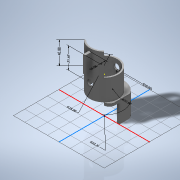
# Autodesk Inventor part: Part1
Saved by Autodesk Inventor 2022 (Build 260153000, 153)
## iProperties
Created: 2021-09-21
Part Number: Part1
Material: Generic
Document SubType Name: Modeling
Designer: WASHINGTON
Density: 1 g/cm^3
Appearance: Default
Author: WASHINGTON
Autodesk Inventor part; units mm, degrees
ref_plane "YZ Plane" through (0, 0, 0) normal (1, 0, 0) x (0, 1, 0)
ref_plane "XZ Plane" through (0, 0, 0) normal (0, 1, 0) x (-1, 0, 0)
sketch "Sketch1" plane through (0, 0, 0) normal (0, 1, 0) x (-1, 0, 0)
  circle A0 centre (0, 0) radius 20.5
  circle A1 centre (0, 0) radius 25
  dimension "d0" = 41
  dimension "d1" = 50
  constraints: 2 centre point, 2 coincident
  measures "d0" diameter of A0
  measures "d1" diameter of A1
extrude "Extrusion1" add sketch "Sketch1" along normal blind 12.5 and the other way blind 25
sketch "Sketch2" plane through (0, 0, 0) normal (0, 0, 1) x (1, 0, 0)
  circle A0 centre (0, 0) radius 5
  dimension "d4" = 10
  constraints: 1 centre point, 1 coincident
  measures "d4" diameter of A0
extrude "Extrusion2" cut sketch "Sketch2" along normal through all both and the other way through all
sketch "Sketch3" plane through (0, -25, 0) normal (0, -1, 0) x (1, 0, 0)
  arc A0 (23.5516, -23.5516) -> (23.5516, 23.5516) centre (0, 0) ccw
  line L0 (0, 0) -> (23.5516, 23.5516) construction
  line L1 (0, 0) -> (33.307, 0) construction
  line L2 (0, 0) -> (23.5516, -23.5516) construction
  circle A1 centre (0, 0) radius 25 construction
  circle A2 centre (0, 0) radius 20.5 construction
  arc A3 (14.4957, -14.4957) -> (14.4957, 14.4957) centre (0, 0) ccw
  line L3 (14.4957, 14.4957) -> (23.5516, 23.5516)
  line L4 (0.0405, -20.5) -> (0.0405, -33.307)
  arc A4 (0.0405, -33.307) -> (23.5516, -23.5516) centre (0, 0) ccw
  arc A5 (0.0405, -20.5) -> (14.4957, -14.4957) centre (0, 0) ccw
  dimension "d7" = 33.307
  dimension "d8" = 45
  dimension "d9" = 90
  dimension "d26" = 12.807
  constraints: 11 point on circle, 10 end point, 4 centre point, 4 coincident, 1 collinear, 1 equal length, 1 horizontal, 1 vertical, 1 other
  measures "d7" radius of A0
  measures "d8" angle of L1 L0
  measures "d9" angle of L2 L0
  measures "d26" distance of L4.start L4.end
extrude "Extrusion3" add sketch "Sketch3" along normal blind 5
sketch "Sketch6" plane through (0, -30, 0) normal (0, -1, 0) x (1, 0, 0)
  arc A0 (0.0405, -20.5) -> (14.4957, 14.4957) centre (0, 0) ccw projected
  line L0 (8.0405, -18.8574) -> (8.0405, -28)
  line L1 (8.0405, -28) -> (0.0405, -28)
  line L2 (0.0405, -28) -> (0.0405, -20.5)
  line L3 (0.0405, -25) -> (0.0405, -20.5) projected
  arc A1 (0.0405, -20.5) -> (8.0405, -18.8574) centre (0, 0) ccw
  dimension "d14" = 8
  dimension "d15" = 42.4957
  constraints: 6 end point, 3 point on circle, 2 parallel, 1 centre point, 1 coincident, 1 horizontal
  measures "d14" distance of L0.end L1.end
  measures "d15" distance from line of A0.end L1
extrude "Extrusion4" add sketch "Sketch6" along normal blind 5
sketch "Sketch7" plane through (0, -30, 0) normal (0, -1, 0) x (1, 0, 0)
  line L0 (0.0405, -28) -> (8.0381, -28) projected
  line L1 (8.0381, -28) -> (18.0381, -28)
  line L2 (18.0381, -28) -> (18.0381, -9.7405)
  line L3 (8.0381, -18.8584) -> (8.0381, -28)
  circle A0 centre (0, 0) radius 20.5
  arc A1 (18.0381, -28) -> (33.3072, 0) centre (0, 0) ccw
  line L4 (33.3072, 0) -> (20.5, 0)
  circle A2 centre (0, 0) radius 20.5 projected
  point P0 (0.0405, -33.307)
  point P1 (8.0405, -18.8574)
  point P2 (8.0381, -18.8584)
  dimension "d19" = 10
  dimension "d22" = 41
  dimension "d23" = 28
  dimension "d24" = 28
  dimension "d25" = 2.4619
  constraints: 6 end point, 5 point on circle, 2 centre point, 2 coincident, 2 horizontal, 1 perpendicular, 1 vertical, 4 other
  measures "d22" diameter of A0
  measures "d23" distance between parallel lines of L4 L0
  measures "d24" distance from line of point (20.5, 0) L0
  measures "d25" distance from line of point (20.5, 0) L2
extrude "Extrusion5" add sketch "Sketch7" along normal blind 23 contours L2 A0 L4 A1
sketch "Sketch8" plane through (8.0405, -30, -28) normal (0, 0, -1) x (-1, 0, 0)
  line L0 (8, -5) -> (0, -5) projected
  line L1 (0, 0) -> (8, 0) projected
  line L2 (8, -5) -> (0, -5)
  line L3 (0, -5) -> (0, 0)
  line L4 (0, 0) -> (8, 0)
  line L5 (8, 0) -> (8, -5)
  point P0 (8.0405, 30)
  constraints: 8 end point, 2 parallel, 1 horizontal, 1 perpendicular
extrude "Extrusion6" add sketch "Sketch8" along normal up to surface round surface about axis through (0, -25, 0) along (0, -1, 0) radius 33.307 far side no
sketch "Sketch9" plane through (0, -53, 0) normal (0, -1, 0) x (1, 0, 0)
  line L0 (0.0405, -25) -> (0.0405, -33.307) projected
  line L1 (0.0405, -33.307) -> (8.0405, -33.307)
  line L2 (8.0405, -33.307) -> (8.0405, -18.8574)
  line L3 (8.0405, -18.8574) -> (0.0405, -18.8574)
  line L4 (0.0405, -18.8574) -> (0.0405, -33.307)
  point P0 (0, 0)
  constraints: 8 end point, 2 parallel, 1 horizontal, 1 perpendicular
extrude "Extrusion7" add sketch "Sketch9" along normal blind 5
sketch "Sketch10" plane through (0, -53, 0) normal (0, -1, 0) x (1, 0, 0)
  line L0 (0.0405, -33.307) -> (8.0405, -33.307) projected
  arc A0 (0.0405, -33.307) -> (23.5516, 23.5516) centre (0, 0) ccw projected
  arc A1 (0.0405, -33.307) -> (33.3068, 0.1051) centre (0, 0) ccw
  line L1 (33.3068, 0.1051) -> (56.6736, 0.1051)
  line L2 (56.6736, 0.1051) -> (0.0405, -55.1449)
  line L3 (0.0405, -55.1449) -> (0.0405, -33.307)
  dimension "d31" = 135.708
  dimension "d32" = 33.4121
  dimension "d33" = 39.9123
  constraints: 6 end point, 3 point on circle, 1 centre point, 1 coincident, 1 horizontal, 1 perpendicular
  measures "d31" angle of L0 L2
  measures "d32" distance between parallel lines of L0 L1
  measures "d33" distance from line of A0.end L2
extrude "Extrusion8" cut sketch "Sketch10" along normal blind 5
sketch "Sketch11" plane through (0, -53, 0) normal (0, -1, 0) x (1, 0, 0)
  arc A0 (0.0405, -33.307) -> (8.0405, -32.3219) centre (0, 0) ccw projected
  line L0 (20.5, 0) -> (33.307, 0) projected
  arc A1 (0.0405, -33.307) -> (33.307, 0) centre (0, 0) ccw
  circle A2 centre (0, 0) radius 20.5 projected
  arc A3 (0.0405, -20.5) -> (20.5, 0) centre (0, 0) ccw
  line L1 (33.307, 0) -> (20.5, 0)
  line L2 (0.0405, -25) -> (0.0405, -33.307) projected
  line L3 (0.0405, -33.307) -> (0.0405, -20.5)
  point P0 (8.0405, -32.3219)
  constraints: 5 point on circle, 4 end point, 2 centre point, 2 coincident, 2 collinear
extrude "Extrusion9" add sketch "Sketch11" along normal blind 5 contours L2 L3 A2 L0 A1 A0
sketch "Sketch12" plane through (0, 0, 0) normal (0, 1, 0) x (-1, 0, 0)
  point P0 (0, 0)
extrude "Extrusion10" cut sketch "Sketch11" along normal blind 5 contours A2
sketch "Sketch13" plane through (0, -58, 0) normal (0, -1, 0) x (1, 0, 0)
  arc A0 (0.0405, -33.307) -> (33.307, 0) centre (0, 0) ccw projected
  line L0 (0.0405, -33.307) -> (0.0405, -20.5)
  line L1 (18.0381, -9.7405) -> (18.0381, -27.9997) projected
  line L2 (18.0381, -27.9997) -> (18.0381, -9.7405)
  arc A1 (0.0405, -20.5) -> (18.0381, -9.7405) centre (0, 0) ccw projected
  arc A2 (0.0405, -20.5) -> (18.0381, -9.7405) centre (0, 0) ccw
  arc A3 (0.0405, -33.307) -> (18.0381, -27.9997) centre (0, 0) ccw projected
  arc A4 (0.0405, -33.307) -> (18.0381, -27.9997) centre (0, 0) ccw
  constraints: 5 point on circle, 4 end point, 2 centre point, 2 coincident, 1 vertical
extrude "Extrusion11" cut sketch "Sketch13" against normal blind 5
sketch "Sketch14" plane through (0, -58, 0) normal (0, -1, 0) x (1, 0, 0)
  line L0 (0.0405, -25) -> (0.0405, -33.307) projected
  line L1 (0.0405, -33.307) -> (0.0405, -20.5)
  circle A0 centre (0, 0) radius 20.5 projected
  line L2 (8.0405, -18.8574) -> (8.0405, -32.3219) projected
  line L3 (8.0405, -32.3219) -> (8.0405, -18.8574)
  arc A1 (0.0405, -20.5) -> (8.0405, -18.8574) centre (0, 0) ccw projected
  arc A2 (8.0405, -18.8574) -> (18.0381, -9.7405) centre (0, 0) ccw projected
  arc A3 (0.0405, -20.5) -> (8.0405, -18.8574) centre (0, 0) ccw
  arc A4 (0.0405, -33.307) -> (8.0405, -32.3219) centre (0, 0) ccw
  constraints: 5 point on circle, 4 end point, 2 centre point, 2 coincident, 1 collinear, 1 vertical
extrude "Extrusion12" add sketch "Sketch14" along normal blind 5 contours L1 A0 L2 A4 L0
sketch "Sketch15" plane through (0, -58, 0) normal (0, -1, 0) x (1, 0, 0)
  line L0 (33.307, 0) -> (20.5, 0) projected
  line L1 (33.307, 0) -> (20.5, 0)
  circle A0 centre (0, 0) radius 20.5 projected
  line L2 (8.0405, -32.3219) -> (8.0405, -18.8574) projected
  line L3 (8.0405, -32.3219) -> (8.0405, -18.8574)
  arc A1 (0.0405, -20.5) -> (8.0405, -18.8574) centre (0, 0) ccw projected
  arc A2 (8.0405, -18.8574) -> (20.5, 0) centre (0, 0) ccw
  arc A3 (8.0405, -32.3219) -> (33.307, 0) centre (0, 0) ccw
  line L4 (8.0405, -32.3219) -> (8.0405, -18.8574)
  constraints: 6 end point, 5 point on circle, 2 centre point, 2 coincident, 2 collinear, 1 horizontal
extrude "Extrusion13" add sketch "Sketch15" along normal blind 5 contours A3 L2 A0 L0
sketch "Sketch16" plane through (0, 0, 0) normal (0, 1, 0) x (-1, 0, 0)
  line L0 (-26.9035, 17.6777) -> (-26.9035, -44.2504)
  line L1 (-26.9035, -44.2504) -> (-40.8771, -44.2504)
  line L2 (-40.8771, -44.2504) -> (-40.8771, 40.313)
  line L3 (-40.8771, 40.313) -> (0, 40.313)
  line L4 (0, 40.313) -> (0, 25.6236)
  line L5 (0, 25.6236) -> (0, 25)
  arc A0 (-0.0405, -25) -> (-17.6777, 17.6777) centre (0, 0) ccw projected
  line L6 (-14.4957, 14.4957) -> (-17.6777, 17.6777) projected
  line L7 (-17.6777, 17.6777) -> (-26.9035, 17.6777)
  arc A1 (0, 25) -> (-17.6777, 17.6777) centre (0, 0) ccw
  constraints: 14 end point, 5 perpendicular, 3 point on circle, 2 point on line, 1 centre point, 1 coincident, 1 vertical
extrude "Extrusion14" cut sketch "Sketch16" against normal through all
fillet "Fillet1" radius 10 1 edges at (26.9035, -27.5, 17.6777)
fillet "Fillet2" radius 10 2 edges at (26.9035, -41.5, -19.636) (26.9035, -27.5, -19.6356)
sketch "Sketch17" plane through (0, 12.5, 0) normal (0, 1, 0) x (1, 0, 0)
  arc A0 (0.0405, 25) -> (17.6777, -17.6777) centre (0, 0) ccw projected
  arc A1 (-18.2219, -17.1162) -> (17.6777, -17.6777) centre (0, 0) ccw
  arc A2 (0.0405, 20.5) -> (14.4957, -14.4957) centre (0, 0) ccw projected
  line L0 (14.4957, -14.4957) -> (17.6777, -17.6777) projected
  arc A3 (-14.4957, -14.4957) -> (14.4957, -14.4957) centre (0, 0) ccw
  line L1 (-15.038, -13.9323) -> (-18.2219, -17.1162)
  line L2 (14.4957, -14.4957) -> (17.6777, -17.6777)
  constraints: 7 point on circle, 4 end point, 2 centre point, 2 coincident, 1 perpendicular
extrude "Extrusion15" add sketch "Sketch17" along normal blind 40
ref_plane "Work Plane1" through (0, 0, 25) normal (0, 0, 1) x (1, 0, 0)
sketch "Sketch18" plane through (0, 0, 25) normal (0, 0, 1) x (1, 0, 0)
  line L0 (-15.038, 52.5) -> (14.4957, 52.5) projected
  line L1 (-20.5, 12.5) -> (20.5, 12.5) projected
  line L2 (-2, 47.5) -> (2, 47.5)
  line L3 (2, 47.5) -> (2, 17.5)
  line L4 (2, 17.5) -> (-2, 17.5)
  line L5 (-2, 17.5) -> (-2, 47.5)
  line L6 (0, 12.5) -> (0, 52.5) construction
  point P0 (0, 0)
  point P1 (-15.038, 12.5)
  point P2 (14.4957, 12.5)
  dimension "d71" = 4
  dimension "d72" = 2
  dimension "d73" = 5
  dimension "d74" = 30
  constraints: 10 end point, 2 parallel, 1 horizontal, 1 midpoint, 1 perpendicular, 1 point on line, 1 vertical
  measures "d71" distance of L2.start L2.end
  measures "d72" distance from line of L6 L2.end
  measures "d73" distance between parallel lines of L0 L2
  measures "d74" distance of L2.end L3.end
extrude "Extrusion16" add sketch "Sketch18" along normal blind 10 and the other way blind 3
sketch "Sketch19" plane through (0, 52.5, 0) normal (0, 1, 0) x (1, 0, 0)
  circle A0 centre (0, 0) radius 22.5
  dimension "d79" = 45
  constraints: 1 centre point, 1 coincident
  measures "d79" diameter of A0
extrude "Extrusion17" cut sketch "Sketch19" against normal through all
body "Solid1"
